Autodesk Fusion 360 part; units mm, degrees
(part 3 of 5)
  spline S734 degree 3 poles (4.2768, -3.4159) (4.27, -4.5634) (4.2456, -6.2234) (4.2225, -7.1047) knots 0 0 0 0 1 1 1 1
  spline S735 degree 3 poles (4.2225, -7.1047) (4.1736, -8.9658) (4.1741, -8.9676) (4.6986, -8.9676) knots 0 0 0 0 1 1 1 1
  spline S736 degree 3 poles (4.6986, -8.9676) (4.9293, -8.9676) (5.068, -8.9294) (5.1437, -8.8451) knots 0 0 0 0 1 1 1 1
  spline S737 degree 3 poles (-7.7375, -7.165) (-7.6403, -7.0562) (-7.6359, -6.8494) (-7.6984, -5.3274) knots 0 0 0 0 1 1 1 1
  spline S738 degree 3 poles (-7.6984, -5.3274) (-7.7797, -3.3444) (-7.7614, -3.2272) (-7.3703, -3.2272) knots 0 0 0 0 1 1 1 1
  spline S739 degree 3 poles (-7.3703, -3.2272) (-7.0455, -3.2272) (-6.9853, -3.3847) (-6.9853, -4.2336) knots 0 0 0 0 1 1 1 1
  spline S740 degree 3 poles (-6.9853, -4.2336) (-6.9853, -5.2382) (-7.167, -5.17) (-4.517, -5.1604) knots 0 0 0 0 1 1 1 1
  spline S741 degree 3 poles (-4.517, -5.1604) (-2.7083, -5.1538) (-2.2947, -5.1343) (-2.1944, -5.051) knots 0 0 0 0 1 1 1 1
  spline S742 degree 3 poles (-2.1944, -5.051) (-2.0819, -4.9577) (-2.0757, -4.8021) (-2.1141, -3.066) knots 0 0 0 0 1 1 1 1
  spline S743 degree 3 poles (-2.1141, -3.066) (-2.1371, -2.0299) (-2.1733, -1.154) (-2.1946, -1.1196) knots 0 0 0 0 1 1 1 1
  spline S744 degree 3 poles (-2.1946, -1.1196) (-2.2168, -1.0837) (-4.8195, -1.0571) (-8.3145, -1.0571) knots 0 0 0 0 1 1 1 1
  spline S745 degree 3 poles (-8.3145, -1.0571) (-13.6654, -1.0571) (-14.4085, -1.0699) (-14.5022, -1.1636) knots 0 0 0 0 1 1 1 1
  spline S746 degree 3 poles (-14.5022, -1.1636) (-14.6184, -1.2797) (-14.6146, -1.6645) (-14.4728, -4.1373) knots 0 0 0 0 1 1 1 1
  spline S747 degree 3 poles (-14.4728, -4.1373) (-14.3583, -6.1352) (-14.267, -6.958) (-14.1447, -7.0942) knots 0 0 0 0 1 1 1 1
  spline S748 degree 3 poles (-14.1447, -7.0942) (-14.0447, -7.2056) (-13.7867, -7.2176) (-11.1229, -7.235) knots 0 0 0 0 1 1 1 1
  spline S749 degree 3 poles (-11.1229, -7.235) (-9.521, -7.2455) (-8.1286, -7.2616) (-8.0287, -7.2708) knots 0 0 0 0 1 1 1 1
  spline S750 degree 3 poles (-8.0287, -7.2708) (-7.9262, -7.2802) (-7.7993, -7.2341) (-7.7375, -7.165) knots 0 0 0 0 1 1 1 1
  spline S751 degree 3 poles (-15.1497, -7.1114) (-15.0136, -6.9753) (-15.0146, -7.1038) (-15.1381, -5.6424) knots 0 0 0 0 1 1 1 1
  spline S752 degree 3 poles (-15.1381, -5.6424) (-15.1934, -4.9878) (-15.2581, -3.964) (-15.2817, -3.3672) knots 0 0 0 0 1 1 1 1
  spline S753 degree 3 poles (-15.2817, -3.3672) (-15.3054, -2.7704) (-15.3347, -2.0537) (-15.3469, -1.7744) knots 0 0 0 0 1 1 1 1
  spline S754 degree 3 poles (-15.3469, -1.7744) (-15.359, -1.4952) (-15.4081, -1.2196) (-15.4559, -1.1619) knots 0 0 0 0 1 1 1 1
  spline S755 degree 3 poles (-15.4559, -1.1619) (-15.5314, -1.071) (-16.0972, -1.0571) (-19.7322, -1.0571) knots 0 0 0 0 1 1 1 1
  spline S756 degree 3 poles (-19.7322, -1.0571) (-23.6509, -1.0571) (-23.9255, -1.065) (-23.9853, -1.1796) knots 0 0 0 0 1 1 1 1
  spline S757 degree 3 poles (-23.9853, -1.1796) (-24.1581, -1.5109) (-23.6522, -6.7547) (-23.4262, -6.9753) knots 0 0 0 0 1 1 1 1
  spline S758 degree 3 poles (-23.4262, -6.9753) (-23.3521, -7.0476) (-22.6326, -7.0805) (-20.1461, -7.1252) knots 0 0 0 0 1 1 1 1
  spline S759 degree 3 poles (-20.1461, -7.1252) (-18.3942, -7.1567) (-16.579, -7.1921) (-16.1123, -7.2039) knots 0 0 0 0 1 1 1 1
  spline S760 degree 3 poles (-16.1123, -7.2039) (-15.4022, -7.2219) (-15.2451, -7.2068) (-15.1497, -7.1114) knots 0 0 0 0 1 1 1 1
  spline S761 degree 3 poles (20.0321, -7.0477) (20.1165, -6.946) (20.2451, -5.9874) (20.3851, -4.4173) knots 0 0 0 0 1 1 1 1
  spline S762 degree 3 poles (20.3851, -4.4173) (20.4607, -3.5699) (20.47, -3.5361) (20.6793, -3.3497) knots 0 0 0 0 1 1 1 1
  spline S763 degree 3 poles (20.6793, -3.3497) (20.8909, -3.1612) (20.914, -3.1572) (21.7814, -3.1572) knots 0 0 0 0 1 1 1 1
  line L87 (21.7814, -3.1572) -> (22.6674, -3.1572)
  line L88 (22.6674, -3.1572) -> (22.9766, -3.4722)
  spline S764 degree 3 poles (22.9766, -3.4722) (23.2635, -3.7646) (23.3116, -3.7873) (23.6454, -3.7873) knots 0 0 0 0 1 1 1 1
  spline S765 degree 3 poles (23.6454, -3.7873) (24.1649, -3.7873) (24.2165, -3.7033) (24.269, -2.7722) knots 0 0 0 0 1 1 1 1
  spline S766 degree 3 poles (24.269, -2.7722) (24.2929, -2.3487) (24.3272, -1.8511) (24.3453, -1.6665) knots 0 0 0 0 1 1 1 1
  spline S767 degree 3 poles (24.3453, -1.6665) (24.4099, -1.008) (24.6837, -1.0571) (20.9465, -1.0571) knots 0 0 0 0 1 1 1 1
  spline S768 degree 3 poles (20.9465, -1.0571) (17.7701, -1.0571) (17.6588, -1.0616) (17.5887, -1.1925) knots 0 0 0 0 1 1 1 1
  spline S769 degree 3 poles (17.5887, -1.1925) (17.5489, -1.267) (17.516, -1.6371) (17.5157, -2.015) knots 0 0 0 0 1 1 1 1
  spline S770 degree 3 poles (17.5157, -2.015) (17.5149, -2.7862) (17.3457, -5.3852) (17.2344, -6.3324) knots 0 0 0 0 1 1 1 1
  spline S771 degree 3 poles (17.2344, -6.3324) (17.1803, -6.7925) (17.1824, -6.9776) (17.2425, -7.05) knots 0 0 0 0 1 1 1 1
  spline S772 degree 3 poles (17.2425, -7.05) (17.3623, -7.1943) (19.9121, -7.1922) (20.0321, -7.0477) knots 0 0 0 0 1 1 1 1
  spline S773 degree 3 poles (27.0719, -6.9725) (28.7644, -6.9359) (29.1939, -6.9073) (29.2848, -6.8252) knots 0 0 0 0 1 1 1 1
  spline S774 degree 3 poles (29.2848, -6.8252) (29.5576, -6.5788) (30.1767, -1.4027) (29.9641, -1.1465) knots 0 0 0 0 1 1 1 1
  spline S775 degree 3 poles (29.9641, -1.1465) (29.9066, -1.0773) (29.3748, -1.0573) (27.6058, -1.0582) knots 0 0 0 0 1 1 1 1
  spline S776 degree 3 poles (27.6058, -1.0582) (26.3464, -1.0587) (25.2763, -1.088) (25.2205, -1.1233) knots 0 0 0 0 1 1 1 1
  spline S777 degree 3 poles (25.2205, -1.1233) (25.1439, -1.1718) (25.1061, -1.4402) (25.0654, -2.2248) knots 0 0 0 0 1 1 1 1
  spline S778 degree 3 poles (25.0654, -2.2248) (25.0016, -3.4565) (24.8292, -5.2439) (24.686, -6.16) knots 0 0 0 0 1 1 1 1
  spline S779 degree 3 poles (24.686, -6.16) (24.5925, -6.7582) (24.5935, -6.8289) (24.6965, -6.9428) knots 0 0 0 0 1 1 1 1
  spline S780 degree 3 poles (24.6965, -6.9428) (24.7589, -7.0117) (24.8463, -7.0568) (24.8908, -7.043) knots 0 0 0 0 1 1 1 1
  spline S781 degree 3 poles (24.8908, -7.043) (24.9353, -7.0292) (25.9168, -6.9975) (27.0719, -6.9725) knots 0 0 0 0 1 1 1 1
  spline S782 degree 3 poles (-24.3456, -6.866) (-24.3039, -6.7882) (-24.2846, -6.7007) (-24.3025, -6.6717) knots 0 0 0 0 1 1 1 1
  spline S783 degree 3 poles (-24.3025, -6.6717) (-24.3372, -6.6155) (-24.5035, -5.3894) (-24.6286, -4.2679) knots 0 0 0 0 1 1 1 1
  spline S784 degree 3 poles (-24.6286, -4.2679) (-24.67, -3.8969) (-24.728, -3.0721) (-24.7576, -2.435) knots 0 0 0 0 1 1 1 1
  spline S785 degree 3 poles (-24.7576, -2.435) (-24.7937, -1.6576) (-24.8414, -1.2404) (-24.9025, -1.1668) knots 0 0 0 0 1 1 1 1
  spline S786 degree 3 poles (-24.9025, -1.1668) (-24.9817, -1.0713) (-25.2907, -1.0571) (-27.2926, -1.0571) knots 0 0 0 0 1 1 1 1
  spline S787 degree 3 poles (-27.2926, -1.0571) (-29.4108, -1.0571) (-29.5968, -1.0667) (-29.6566, -1.1796) knots 0 0 0 0 1 1 1 1
  spline S788 degree 3 poles (-29.6566, -1.1796) (-29.8456, -1.5361) (-29.2581, -6.514) (-28.9925, -6.8075) knots 0 0 0 0 1 1 1 1
  spline S789 degree 3 poles (-28.9925, -6.8075) (-28.871, -6.9417) (-28.7554, -6.9479) (-25.5564, -6.9919) knots 0 0 0 0 1 1 1 1
  spline S790 degree 3 poles (-25.5564, -6.9919) (-24.4807, -7.0066) (-24.4173, -7.0001) (-24.3456, -6.866) knots 0 0 0 0 1 1 1 1
  spline S791 degree 3 poles (-29.9974, -6.7448) (-29.8983, -6.6353) (-29.8967, -6.5674) (-29.9829, -6.115) knots 0 0 0 0 1 1 1 1
  spline S792 degree 3 poles (-29.9829, -6.115) (-30.1257, -5.3656) (-30.35, -3.4788) (-30.4384, -2.2838) knots 0 0 0 0 1 1 1 1
  spline S793 degree 3 poles (-30.4384, -2.2838) (-30.481, -1.7072) (-30.5492, -1.1953) (-30.5899, -1.1462) knots 0 0 0 0 1 1 1 1
  spline S794 degree 3 poles (-30.5899, -1.1462) (-30.6927, -1.0223) (-33.6594, -1.0176) (-33.7829, -1.1411) knots 0 0 0 0 1 1 1 1
  spline S795 degree 3 poles (-33.7829, -1.1411) (-33.9031, -1.2613) (-33.8872, -1.8592) (-33.7257, -3.2908) knots 0 0 0 0 1 1 1 1
  spline S796 degree 3 poles (-33.7257, -3.2908) (-33.5508, -4.8422) (-33.2687, -6.4463) (-33.1506, -6.5614) knots 0 0 0 0 1 1 1 1
  spline S797 degree 3 poles (-33.1506, -6.5614) (-33.0737, -6.6365) (-32.3628, -6.7147) (-30.7867, -6.8216) knots 0 0 0 0 1 1 1 1
  spline S798 degree 3 poles (-30.7867, -6.8216) (-30.6135, -6.8334) (-30.3899, -6.8485) (-30.29, -6.8552) knots 0 0 0 0 1 1 1 1
  spline S799 degree 3 poles (-30.29, -6.8552) (-30.1901, -6.8619) (-30.0584, -6.8122) (-29.9974, -6.7448) knots 0 0 0 0 1 1 1 1
  spline S800 degree 3 poles (31.1807, -6.7419) (31.275, -6.6475) (31.5379, -5.2425) (31.6615, -4.1723) knots 0 0 0 0 1 1 1 1
  spline S801 degree 3 poles (31.6615, -4.1723) (31.7475, -3.4274) (31.7585, -3.3948) (31.9975, -3.1747) knots 0 0 0 0 1 1 1 1
  line L89 (31.9975, -3.1747) -> (32.2445, -2.9472)
  line L90 (32.2445, -2.9472) -> (33.0281, -2.9472)
  spline S802 degree 3 poles (33.0281, -2.9472) (34.0757, -2.9472) (34.0873, -2.9374) (34.1613, -1.9839) knots 0 0 0 0 1 1 1 1
  spline S803 degree 3 poles (34.1613, -1.9839) (34.1919, -1.5888) (34.1907, -1.2186) (34.1586, -1.1613) knots 0 0 0 0 1 1 1 1
  spline S804 degree 3 poles (34.1586, -1.1613) (34.0766, -1.0147) (31.0188, -1.0054) (30.8728, -1.1513) knots 0 0 0 0 1 1 1 1
  spline S805 degree 3 poles (30.8728, -1.1513) (30.8151, -1.209) (30.7711, -1.4464) (30.7592, -1.7638) knots 0 0 0 0 1 1 1 1
  spline S806 degree 3 poles (30.7592, -1.7638) (30.7294, -2.5612) (30.4864, -4.8147) (30.3292, -5.7512) knots 0 0 0 0 1 1 1 1
  spline S807 degree 3 poles (30.3292, -5.7512) (30.1516, -6.8092) (30.1825, -6.8934) (30.732, -6.8498) knots 0 0 0 0 1 1 1 1
  spline S808 degree 3 poles (30.732, -6.8498) (30.9355, -6.8337) (31.1374, -6.7851) (31.1807, -6.7419) knots 0 0 0 0 1 1 1 1
  line L91 (31.1807, -6.7419) -> (31.1807, -6.7419)
  spline S809 degree 3 poles (33.4591, -6.5656) (33.5108, -6.5139) (33.6498, -5.8956) (33.768, -5.1916) knots 0 0 0 0 1 1 1 1
  spline S810 degree 3 poles (33.768, -5.1916) (33.9788, -3.9355) (33.9803, -3.9092) (33.8502, -3.7791) knots 0 0 0 0 1 1 1 1
  spline S811 degree 3 poles (33.8502, -3.7791) (33.7337, -3.6626) (33.6513, -3.6521) (33.1716, -3.6926) knots 0 0 0 0 1 1 1 1
  spline S812 degree 3 poles (33.1716, -3.6926) (32.8714, -3.718) (32.5872, -3.7772) (32.5402, -3.8242) knots 0 0 0 0 1 1 1 1
  spline S813 degree 3 poles (32.5402, -3.8242) (32.4932, -3.8713) (32.4163, -4.2051) (32.3693, -4.566) knots 0 0 0 0 1 1 1 1
  spline S814 degree 3 poles (32.3693, -4.566) (32.3223, -4.927) (32.2348, -5.5153) (32.1749, -5.8734) knots 0 0 0 0 1 1 1 1
  spline S815 degree 3 poles (32.1749, -5.8734) (32.0308, -6.7344) (32.051, -6.761) (32.8072, -6.7027) knots 0 0 0 0 1 1 1 1
  spline S816 degree 3 poles (32.8072, -6.7027) (33.1268, -6.678) (33.4052, -6.6195) (33.4591, -6.5656) knots 0 0 0 0 1 1 1 1
  spline S817 degree 3 poles (23.8843, -5.9952) (23.925, -5.9462) (23.9908, -5.6461) (24.0307, -5.3283) knots 0 0 0 0 1 1 1 1
  spline S818 degree 3 poles (24.0307, -5.3283) (24.123, -4.5919) (24.0582, -4.4907) (23.519, -4.5295) knots 0 0 0 0 1 1 1 1
  spline S819 degree 3 poles (23.519, -4.5295) (23.3207, -4.5438) (23.1213, -4.5953) (23.0758, -4.6439) knots 0 0 0 0 1 1 1 1
  spline S820 degree 3 poles (23.0758, -4.6439) (23.0304, -4.6925) (22.9593, -5.0001) (22.9177, -5.3274) knots 0 0 0 0 1 1 1 1
  spline S821 degree 3 poles (22.9177, -5.3274) (22.8494, -5.8659) (22.8539, -5.9324) (22.9659, -6.0277) knots 0 0 0 0 1 1 1 1
  spline S822 degree 3 poles (22.9659, -6.0277) (23.1151, -6.1546) (23.7713, -6.1315) (23.8843, -5.9952) knots 0 0 0 0 1 1 1 1
  spline S823 degree 3 poles (-28.6306, -0.203) (-28.578, -0.1505) (-28.5466, 0.1107) (-28.5466, 0.4945) knots 0 0 0 0 1 1 1 1
  spline S824 degree 3 poles (-28.5466, 0.4945) (-28.5466, 1.0295) (-28.5639, 1.1174) (-28.682, 1.1806) knots 0 0 0 0 1 1 1 1
  spline S825 degree 3 poles (-28.682, 1.1806) (-28.7669, 1.226) (-29.6198, 1.2531) (-30.9691, 1.2531) knots 0 0 0 0 1 1 1 1
  spline S826 degree 3 poles (-30.9691, 1.2531) (-33.5287, 1.2531) (-33.3769, 1.302) (-33.3769, 0.4772) knots 0 0 0 0 1 1 1 1
  spline S827 degree 3 poles (-33.3769, 0.4772) (-33.3769, 0.0758) (-33.348, -0.0959) (-33.2669, -0.177) knots 0 0 0 0 1 1 1 1
  spline S828 degree 3 poles (-33.2669, -0.177) (-33.1715, -0.2724) (-32.8616, -0.287) (-30.9357, -0.287) knots 0 0 0 0 1 1 1 1
  spline S829 degree 3 poles (-30.9357, -0.287) (-29.3015, -0.287) (-28.6924, -0.2648) (-28.6306, -0.203) knots 0 0 0 0 1 1 1 1
  spline S830 degree 3 poles (-19.6, -0.203) (-19.4866, -0.0896) (-19.4866, 1.0556) (-19.6, 1.1691) knots 0 0 0 0 1 1 1 1
  spline S831 degree 3 poles (-19.6, 1.1691) (-19.6634, 1.2324) (-20.6523, 1.2531) (-23.6213, 1.2531) knots 0 0 0 0 1 1 1 1
  line L92 (-23.6213, 1.2531) -> (-27.5586, 1.2531)
  line L93 (-27.5586, 1.2531) -> (-27.6676, 1.0975)
  spline S832 degree 3 poles (-27.6676, 1.0975) (-27.7408, 0.9929) (-27.7765, 0.7824) (-27.7765, 0.4554) knots 0 0 0 0 1 1 1 1
  spline S833 degree 3 poles (-27.7765, 0.4554) (-27.7765, -0.3571) (-28.1691, -0.287) (-23.6144, -0.287) knots 0 0 0 0 1 1 1 1
  spline S834 degree 3 poles (-23.6144, -0.287) (-20.6508, -0.287) (-19.6634, -0.2664) (-19.6, -0.203) knots 0 0 0 0 1 1 1 1
  spline S835 degree 3 poles (-4.1031, -0.1712) (-3.9171, -0.0028) (-3.9167, 0.9685) (-4.1026, 1.1368) knots 0 0 0 0 1 1 1 1
  spline S836 degree 3 poles (-4.1026, 1.1368) (-4.2193, 1.2424) (-4.8358, 1.2521) (-11.382, 1.2517) knots 0 0 0 0 1 1 1 1
  line L94 (-11.382, 1.2517) -> (-18.5339, 1.2512)
  line L95 (-18.5339, 1.2512) -> (-18.6402, 1.0889)
  spline S837 degree 3 poles (-18.6402, 1.0889) (-18.7826, 0.8717) (-18.7685, 0.0077) (-18.6199, -0.1645) knots 0 0 0 0 1 1 1 1
  spline S838 degree 3 poles (-18.6199, -0.1645) (-18.5205, -0.2797) (-18.0872, -0.287) (-11.3726, -0.287) knots 0 0 0 0 1 1 1 1
  spline S839 degree 3 poles (-11.3726, -0.287) (-4.8256, -0.287) (-4.2204, -0.2774) (-4.103, -0.1712) knots 0 0 0 0 1 1 1 1
  line L96 (-4.103, -0.1712) -> (-4.1031, -0.1712)
  spline S840 degree 3 poles (13.232, -0.203) (13.3455, -0.0896) (13.3455, 1.0556) (13.232, 1.1691) knots 0 0 0 0 1 1 1 1
  spline S841 degree 3 poles (13.232, 1.1691) (13.1062, 1.2948) (-3.0167, 1.2906) (-3.1211, 1.1648) knots 0 0 0 0 1 1 1 1
  spline S842 degree 3 poles (-3.1211, 1.1648) (-3.2358, 1.0267) (-3.2513, -0.042) (-3.1405, -0.1754) knots 0 0 0 0 1 1 1 1
  spline S843 degree 3 poles (-3.1405, -0.1754) (-3.0567, -0.2764) (-2.2771, -0.287) (5.0501, -0.287) knots 0 0 0 0 1 1 1 1
  spline S844 degree 3 poles (5.0501, -0.287) (11.2551, -0.287) (13.1676, -0.2674) (13.232, -0.203) knots 0 0 0 0 1 1 1 1
  spline S845 degree 3 poles (20.2324, -0.203) (20.2847, -0.1507) (20.3164, 0.1081) (20.3164, 0.483) knots 0 0 0 0 1 1 1 1
  spline S846 degree 3 poles (20.3164, 0.483) (20.3164, 0.8579) (20.2847, 1.1167) (20.2324, 1.1691) knots 0 0 0 0 1 1 1 1
  spline S847 degree 3 poles (20.2324, 1.1691) (20.1698, 1.2317) (19.4099, 1.2531) (17.2453, 1.2531) knots 0 0 0 0 1 1 1 1
  spline S848 degree 3 poles (17.2453, 1.2531) (13.8367, 1.2531) (14.0861, 1.3129) (14.0861, 0.4952) knots 0 0 0 0 1 1 1 1
  spline S849 degree 3 poles (14.0861, 0.4952) (14.0861, -0.3526) (13.8223, -0.287) (17.2331, -0.287) knots 0 0 0 0 1 1 1 1
  spline S850 degree 3 poles (17.2331, -0.287) (19.4072, -0.287) (20.1698, -0.2657) (20.2324, -0.203) knots 0 0 0 0 1 1 1 1
  spline S851 degree 3 poles (28.0989, -0.1712) (28.2013, -0.0785) (28.2269, 0.05) (28.2269, 0.4708) knots 0 0 0 0 1 1 1 1
  spline S852 degree 3 poles (28.2269, 0.4708) (28.2269, 1.3245) (28.5557, 1.2531) (24.6249, 1.2531) knots 0 0 0 0 1 1 1 1
  spline S853 degree 3 poles (24.6249, 1.2531) (22.0968, 1.2531) (21.2335, 1.2321) (21.1705, 1.1691) knots 0 0 0 0 1 1 1 1
  spline S854 degree 3 poles (21.1705, 1.1691) (21.1182, 1.1167) (21.0865, 0.8579) (21.0865, 0.483) knots 0 0 0 0 1 1 1 1
  spline S855 degree 3 poles (21.0865, 0.483) (21.0865, 0.1081) (21.1182, -0.1507) (21.1705, -0.203) knots 0 0 0 0 1 1 1 1
  spline S856 degree 3 poles (21.1705, -0.203) (21.2335, -0.266) (22.0941, -0.287) (24.6127, -0.287) knots 0 0 0 0 1 1 1 1
  spline S857 degree 3 poles (24.6127, -0.287) (27.6393, -0.287) (27.9835, -0.2756) (28.0989, -0.1712) knots 0 0 0 0 1 1 1 1
  spline S858 degree 3 poles (33.5592, -0.1712) (33.6616, -0.0785) (33.6873, 0.05) (33.6873, 0.4708) knots 0 0 0 0 1 1 1 1
  spline S859 degree 3 poles (33.6873, 0.4708) (33.6873, 1.3036) (33.8403, 1.2531) (31.3193, 1.2531) knots 0 0 0 0 1 1 1 1
  spline S860 degree 3 poles (31.3193, 1.2531) (28.7831, 1.2531) (28.927, 1.2986) (28.927, 0.4952) knots 0 0 0 0 1 1 1 1
  spline S861 degree 3 poles (28.927, 0.4952) (28.927, -0.3376) (28.774, -0.287) (31.295, -0.287) knots 0 0 0 0 1 1 1 1
  spline S862 degree 3 poles (31.295, -0.287) (33.1845, -0.287) (33.446, -0.2737) (33.5592, -0.1712) knots 0 0 0 0 1 1 1 1
  spline S863 degree 3 poles (22.4173, 2.1644) (22.4596, 2.2435) (22.46, 2.6704) (22.4183, 3.3284) knots 0 0 0 0 1 1 1 1
  line L97 (22.4183, 3.3284) -> (22.3525, 4.3676)
  line L98 (22.3525, 4.3676) -> (22.5733, 4.5954)
  spline S864 degree 3 poles (22.5733, 4.5954) (22.7891, 4.8181) (22.808, 4.8233) (23.4019, 4.8233) knots 0 0 0 0 1 1 1 1
  spline S865 degree 3 poles (23.4019, 4.8233) (23.8371, 4.8233) (24.0327, 4.8511) (24.0909, 4.9212) knots 0 0 0 0 1 1 1 1
  spline S866 degree 3 poles (24.0909, 4.9212) (24.2074, 5.0616) (24.1117, 5.9094) (23.9648, 6.037) knots 0 0 0 0 1 1 1 1
  spline S867 degree 3 poles (23.9648, 6.037) (23.8721, 6.1177) (23.1892, 6.1423) (20.1678, 6.1741) knots 0 0 0 0 1 1 1 1
  spline S868 degree 3 poles (20.1678, 6.1741) (17.4864, 6.2023) (16.4623, 6.1914) (16.405, 6.1341) knots 0 0 0 0 1 1 1 1
  spline S869 degree 3 poles (16.405, 6.1341) (16.3617, 6.0908) (16.3263, 5.846) (16.3263, 5.5902) knots 0 0 0 0 1 1 1 1
  spline S870 degree 3 poles (16.3263, 5.5902) (16.3263, 4.9083) (16.3284, 4.9073) (17.7234, 4.8861) knots 0 0 0 0 1 1 1 1
  line L99 (17.7234, 4.8861) -> (18.8755, 4.8686)
  line L100 (18.8755, 4.8686) -> (19.1134, 4.6505)
  line L101 (19.1134, 4.6505) -> (19.3513, 4.4325)
  line L102 (19.3513, 4.4325) -> (19.388, 3.3503)
  spline S871 degree 3 poles (19.388, 3.3503) (19.4082, 2.7551) (19.4528, 2.2137) (19.4872, 2.1472) knots 0 0 0 0 1 1 1 1
  spline S872 degree 3 poles (19.4872, 2.1472) (19.5425, 2.0401) (19.7011, 2.024) (20.8607, 2.0071) knots 0 0 0 0 1 1 1 1
  spline S873 degree 3 poles (20.8607, 2.0071) (21.5817, 1.9967) (22.2119, 1.9997) (22.2611, 2.0138) knots 0 0 0 0 1 1 1 1
  spline S874 degree 3 poles (22.2611, 2.0138) (22.3103, 2.028) (22.3806, 2.0958) (22.4174, 2.1644) knots 0 0 0 0 1 1 1 1
  line L103 (22.4174, 2.1644) -> (22.4173, 2.1644)
  spline S875 degree 3 poles (34.1084, 2.1407) (34.2143, 2.2533) (34.221, 2.3495) (34.166, 2.9682) knots 0 0 0 0 1 1 1 1
  spline S876 degree 3 poles (34.166, 2.9682) (34.0827, 3.9038) (34.0917, 3.8969) (32.9358, 3.9057) knots 0 0 0 0 1 1 1 1
  spline S877 degree 3 poles (32.9358, 3.9057) (32.4443, 3.9094) (31.6422, 3.9328) (31.1534, 3.9575) knots 0 0 0 0 1 1 1 1
  spline S878 degree 3 poles (31.1534, 3.9575) (30.2969, 4.0009) (30.2579, 4.0097) (30.0759, 4.1996) knots 0 0 0 0 1 1 1 1
  spline S879 degree 3 poles (30.0759, 4.1996) (29.9048, 4.3783) (29.8748, 4.4938) (29.7558, 5.4326) knots 0 0 0 0 1 1 1 1
  spline S880 degree 3 poles (29.7558, 5.4326) (29.5711, 6.8889) (29.4243, 7.6385) (29.2958, 7.781) knots 0 0 0 0 1 1 1 1
  spline S881 degree 3 poles (29.2958, 7.781) (29.1413, 7.9523) (28.5701, 7.9493) (28.4137, 7.7764) knots 0 0 0 0 1 1 1 1
  spline S882 degree 3 poles (28.4137, 7.7764) (28.3095, 7.6613) (28.308, 7.6004) (28.3979, 7.1289) knots 0 0 0 0 1 1 1 1
  spline S883 degree 3 poles (28.3979, 7.1289) (28.4524, 6.8426) (28.5523, 6.1265) (28.6199, 5.5376) knots 0 0 0 0 1 1 1 1
  line L104 (28.6199, 5.5376) -> (28.7428, 4.4668)
  line L105 (28.7428, 4.4668) -> (28.5185, 4.2425)
  line L106 (28.5185, 4.2425) -> (28.2942, 4.0182)
  line L107 (28.2942, 4.0182) -> (25.7929, 4.0419)
  spline S884 degree 3 poles (25.7929, 4.0419) (23.4252, 4.0643) (23.2876, 4.0587) (23.2157, 3.9369) knots 0 0 0 0 1 1 1 1
  spline S885 degree 3 poles (23.2157, 3.9369) (23.0937, 3.7299) (23.192, 2.1733) (23.3336, 2.0699) knots 0 0 0 0 1 1 1 1
  spline S886 degree 3 poles (23.3336, 2.0699) (23.417, 2.009) (24.7902, 1.9913) (28.717, 2.0007) knots 0 0 0 0 1 1 1 1
  spline S887 degree 3 poles (28.717, 2.0007) (33.7156, 2.0126) (33.9947, 2.0198) (34.1084, 2.1407) knots 0 0 0 0 1 1 1 1
  spline S888 degree 3 poles (-26.8081, 2.1141) (-26.7666, 2.1641) (-26.6984, 2.6918) (-26.6565, 3.2867) knots 0 0 0 0 1 1 1 1
  spline S889 degree 3 poles (-26.6565, 3.2867) (-26.5527, 4.7638) (-26.4054, 6.1913) (-26.2711, 7.0222) knots 0 0 0 0 1 1 1 1
  spline S890 degree 3 poles (-26.2711, 7.0222) (-26.123, 7.9391) (-26.1054, 7.9221) (-27.192, 7.9108) knots 0 0 0 0 1 1 1 1
  spline S891 degree 3 poles (-27.192, 7.9108) (-28.2199, 7.9001) (-29.2313, 7.8545) (-31.3456, 7.7237) knots 0 0 0 0 1 1 1 1
  spline S892 degree 3 poles (-31.3456, 7.7237) (-32.7876, 7.6344) (-33.0059, 7.6056) (-33.123, 7.4884) knots 0 0 0 0 1 1 1 1
  spline S893 degree 3 poles (-33.123, 7.4884) (-33.3262, 7.2852) (-33.6509, 5.1938) (-33.8931, 2.5274) knots 0 0 0 0 1 1 1 1
  spline S894 degree 3 poles (-33.8931, 2.5274) (-33.9414, 1.9957) (-34.1365, 2.0231) (-30.3003, 2.0231) knots 0 0 0 0 1 1 1 1
  spline S895 degree 3 poles (-30.3003, 2.0231) (-27.5829, 2.0231) (-26.8682, 2.0417) (-26.8081, 2.1141) knots 0 0 0 0 1 1 1 1
  spline S896 degree 3 poles (-21.1271, 2.1269) (-21.0745, 2.1903) (-21.0284, 2.5509) (-21.0087, 3.0545) knots 0 0 0 0 1 1 1 1
  spline S897 degree 3 poles (-21.0087, 3.0545) (-20.9909, 3.5075) (-20.9334, 4.3507) (-20.8808, 4.9283) knots 0 0 0 0 1 1 1 1
  spline S898 degree 3 poles (-20.8808, 4.9283) (-20.8029, 5.783) (-20.8019, 5.9954) (-20.875, 6.0702) knots 0 0 0 0 1 1 1 1
  spline S899 degree 3 poles (-20.875, 6.0702) (-20.9244, 6.1207) (-21.218, 6.2498) (-21.5275, 6.3569) knots 0 0 0 0 1 1 1 1
  spline S900 degree 3 poles (-21.5275, 6.3569) (-22.4234, 6.6671) (-23.1908, 7.1243) (-23.8563, 7.7441) knots 0 0 0 0 1 1 1 1
  spline S901 degree 3 poles (-23.8563, 7.7441) (-24.0886, 7.9604) (-24.1292, 7.9723) (-24.6388, 7.9729) knots 0 0 0 0 1 1 1 1
  spline S902 degree 3 poles (-24.6388, 7.9729) (-25.0146, 7.9733) (-25.2068, 7.9431) (-25.2774, 7.8724) knots 0 0 0 0 1 1 1 1
  spline S903 degree 3 poles (-25.2774, 7.8724) (-25.5207, 7.6291) (-26.0597, 2.4868) (-25.8775, 2.1465) knots 0 0 0 0 1 1 1 1
  spline S904 degree 3 poles (-25.8775, 2.1465) (-25.8165, 2.0325) (-25.637, 2.0231) (-23.5124, 2.0231) knots 0 0 0 0 1 1 1 1
  spline S905 degree 3 poles (-23.5124, 2.0231) (-21.5661, 2.0231) (-21.2, 2.039) (-21.1271, 2.1269) knots 0 0 0 0 1 1 1 1
  spline S906 degree 3 poles (-9.7877, 2.1253) (-9.6924, 2.2403) (-9.6684, 2.6014) (-9.6131, 4.7533) knots 0 0 0 0 1 1 1 1
  spline S907 degree 3 poles (-9.6131, 4.7533) (-9.5919, 5.5811) (-9.5545, 6.6089) (-9.5302, 7.0373) knots 0 0 0 0 1 1 1 1
  spline S908 degree 3 poles (-9.5302, 7.0373) (-9.5058, 7.4657) (-9.5066, 7.8988) (-9.532, 7.9998) knots 0 0 0 0 1 1 1 1
  line L108 (-9.532, 7.9998) -> (-9.5781, 8.1835)
  line L109 (-9.5781, 8.1835) -> (-10.9843, 8.1835)
  line L110 (-10.9843, 8.1835) -> (-12.3905, 8.1835)
  line L111 (-12.3905, 8.1835) -> (-13.1502, 7.7258)
  spline S909 degree 3 poles (-13.1502, 7.7258) (-15.0654, 6.5718) (-16.851, 6.0216) (-18.851, 5.9689) knots 0 0 0 0 1 1 1 1
  spline S910 degree 3 poles (-18.851, 5.9689) (-19.6852, 5.947) (-19.9174, 5.9194) (-19.9805, 5.835) knots 0 0 0 0 1 1 1 1
  spline S911 degree 3 poles (-19.9805, 5.835) (-20.119, 5.6496) (-20.3179, 2.3674) (-20.2041, 2.1456) knots 0 0 0 0 1 1 1 1
  spline S912 degree 3 poles (-20.2041, 2.1456) (-20.1451, 2.0306) (-19.8261, 2.0231) (-15.0069, 2.0231) knots 0 0 0 0 1 1 1 1
  spline S913 degree 3 poles (-15.0069, 2.0231) (-10.5907, 2.0231) (-9.8608, 2.0374) (-9.7878, 2.1253) knots 0 0 0 0 1 1 1 1
  line L112 (-9.7878, 2.1253) -> (-9.7877, 2.1253)
  spline S914 degree 3 poles (1.6085, 5.0269) (1.6255, 7.7783) (1.6178, 8.0058) (1.5035, 8.1321) knots 0 0 0 0 1 1 1 1
  spline S915 degree 3 poles (1.5035, 8.1321) (1.3831, 8.2653) (1.266, 8.2678) (-3.5658, 8.2402) knots 0 0 0 0 1 1 1 1
  spline S916 degree 3 poles (-3.5658, 8.2402) (-7.2678, 8.219) (-8.5372, 8.1908) (-8.6128, 8.1281) knots 0 0 0 0 1 1 1 1
  spline S917 degree 3 poles (-8.6128, 8.1281) (-8.7257, 8.0344) (-8.7633, 7.4807) (-8.8769, 4.241) knots 0 0 0 0 1 1 1 1
  spline S918 degree 3 poles (-8.8769, 4.241) (-8.9238, 2.9036) (-8.9224, 2.2511) (-8.8726, 2.1579) knots 0 0 0 0 1 1 1 1
  spline S919 degree 3 poles (-8.8726, 2.1579) (-8.8016, 2.0253) (-8.6826, 2.0226) (-3.6048, 2.0402) knots 0 0 0 0 1 1 1 1
  line L113 (-3.6048, 2.0402) -> (1.5903, 2.0581)
  line L114 (1.5903, 2.0581) -> (1.6085, 5.0269)
  spline S920 degree 3 poles (18.6197, 2.1106) (18.6631, 2.1645) (18.6762, 2.527) (18.6538, 3.0534) knots 0 0 0 0 1 1 1 1
  spline S921 degree 3 poles (18.6538, 3.0534) (18.6251, 3.7257) (18.5926, 3.9311) (18.5021, 4.013) knots 0 0 0 0 1 1 1 1
  spline S922 degree 3 poles (18.5021, 4.013) (18.4037, 4.1021) (17.8885, 4.1187) (14.968, 4.127) knots 0 0 0 0 1 1 1 1
  line L115 (14.968, 4.127) -> (11.5491, 4.1367)
  line L116 (11.5491, 4.1367) -> (11.2957, 4.369)
  line L117 (11.2957, 4.369) -> (11.0422, 4.6013)
  line L118 (11.0422, 4.6013) -> (11.0171, 5.4298)
  spline S923 degree 3 poles (11.0171, 5.4298) (10.9981, 6.0529) (10.9649, 6.2888) (10.883, 6.3809) knots 0 0 0 0 1 1 1 1
  spline S924 degree 3 poles (10.883, 6.3809) (10.7824, 6.4941) (10.5355, 6.5034) (7.6138, 6.5034) knots 0 0 0 0 1 1 1 1
  spline S925 degree 3 poles (7.6138, 6.5034) (5.2491, 6.5034) (4.4323, 6.4823) (4.3695, 6.4194) knots 0 0 0 0 1 1 1 1
  spline S926 degree 3 poles (4.3695, 6.4194) (4.3233, 6.3732) (4.285, 6.1763) (4.2844, 5.9819) knots 0 0 0 0 1 1 1 1
  spline S927 degree 3 poles (4.2844, 5.9819) (4.2831, 5.4971) (4.1645, 5.2839) (3.8813, 5.2564) knots 0 0 0 0 1 1 1 1
  spline S928 degree 3 poles (3.8813, 5.2564) (3.5685, 5.226) (3.5438, 5.3244) (3.4919, 6.8096) knots 0 0 0 0 1 1 1 1
  spline S929 degree 3 poles (3.4919, 6.8096) (3.465, 7.5816) (3.4176, 8.0977) (3.3682, 8.1571) knots 0 0 0 0 1 1 1 1
  spline S930 degree 3 poles (3.3682, 8.1571) (3.2729, 8.272) (2.727, 8.2861) (2.5268, 8.1789) knots 0 0 0 0 1 1 1 1
  spline S931 degree 3 poles (2.5268, 8.1789) (2.3907, 8.1061) (2.3877, 8.0345) (2.3993, 5.1512) knots 0 0 0 0 1 1 1 1
  spline S932 degree 3 poles (2.3993, 5.1512) (2.4068, 3.2866) (2.4372, 2.1659) (2.4818, 2.1106) knots 0 0 0 0 1 1 1 1
  spline S933 degree 3 poles (2.4818, 2.1106) (2.5376, 2.0415) (4.2365, 2.0231) (10.5508, 2.0231) knots 0 0 0 0 1 1 1 1
  spline S934 degree 3 poles (10.5508, 2.0231) (16.8652, 2.0231) (18.564, 2.0415) (18.6197, 2.1106) knots 0 0 0 0 1 1 1 1
  spline S935 degree 3 poles (27.8342, 4.8848) (27.9465, 5.0088) (27.943, 5.0877) (27.7727, 6.2674) knots 0 0 0 0 1 1 1 1
  spline S936 degree 3 poles (27.7727, 6.2674) (27.5422, 7.8648) (27.5383, 7.8746) (27.1107, 7.9314) knots 0 0 0 0 1 1 1 1
  spline S937 degree 3 poles (27.1107, 7.9314) (26.7193, 7.9833) (26.568, 7.9405) (26.5113, 7.7618) knots 0 0 0 0 1 1 1 1
  spline S938 degree 3 poles (26.5113, 7.7618) (26.4888, 7.691) (26.5348, 7.1505) (26.6135, 6.5607) knots 0 0 0 0 1 1 1 1
  spline S939 degree 3 poles (26.6135, 6.5607) (26.6921, 5.9709) (26.7742, 5.355) (26.7958, 5.192) knots 0 0 0 0 1 1 1 1
  spline S940 degree 3 poles (26.7958, 5.192) (26.8423, 4.841) (26.9555, 4.7583) (27.3935, 4.7554) knots 0 0 0 0 1 1 1 1
  spline S941 degree 3 poles (27.3935, 4.7554) (27.6213, 4.7539) (27.7499, 4.7917) (27.8342, 4.8848) knots 0 0 0 0 1 1 1 1
  spline S942 degree 3 poles (25.9775, 4.9171) (26.0906, 5.0534) (25.7938, 7.5275) (25.6255, 7.851) knots 0 0 0 0 1 1 1 1
  spline S943 degree 3 poles (25.6255, 7.851) (25.5759, 7.9464) (25.4714, 7.9735) (25.1528, 7.9735) knots 0 0 0 0 1 1 1 1
  spline S944 degree 3 poles (25.1528, 7.9735) (24.6167, 7.9735) (24.5566, 7.901) (24.6495, 7.3664) knots 0 0 0 0 1 1 1 1
  spline S945 degree 3 poles (24.6495, 7.3664) (24.6885, 7.142) (24.7699, 6.5196) (24.8304, 5.9833) knots 0 0 0 0 1 1 1 1
  spline S946 degree 3 poles (24.8304, 5.9833) (24.8909, 5.447) (24.9749, 4.9666) (25.0171, 4.9158) knots 0 0 0 0 1 1 1 1
  spline S947 degree 3 poles (25.0171, 4.9158) (25.1211, 4.7905) (25.8733, 4.7916) (25.9775, 4.9171) knots 0 0 0 0 1 1 1 1
  spline S948 degree 3 poles (13.8751, 4.9972) (13.9663, 5.107) (13.941, 5.8339) (13.7973, 7.235) knots 0 0 0 0 1 1 1 1
  spline S949 degree 3 poles (13.7973, 7.235) (13.7088, 8.0986) (13.6674, 8.1835) (13.3344, 8.1835) knots 0 0 0 0 1 1 1 1
  spline S950 degree 3 poles (13.3344, 8.1835) (12.9522, 8.1835) (12.616, 8.5288) (12.616, 8.9211) knots 0 0 0 0 1 1 1 1
  spline S951 degree 3 poles (12.616, 8.9211) (12.616, 9.0807) (12.582, 9.4762) (12.5404, 9.8) knots 0 0 0 0 1 1 1 1
  spline S952 degree 3 poles (12.5404, 9.8) (12.4319, 10.6454) (12.4535, 10.6337) (11.0121, 10.6337) knots 0 0 0 0 1 1 1 1
  spline S953 degree 3 poles (11.0121, 10.6337) (10.1968, 10.6337) (9.8184, 10.6083) (9.7598, 10.5496) knots 0 0 0 0 1 1 1 1
  spline S954 degree 3 poles (9.7598, 10.5496) (9.7069, 10.4968) (9.6758, 10.2327) (9.6758, 9.8376) knots 0 0 0 0 1 1 1 1
  spline S955 degree 3 poles (9.6758, 9.8376) (9.6758, 8.9934) (9.7134, 8.9535) (10.5118, 8.9535) knots 0 0 0 0 1 1 1 1
  spline S956 degree 3 poles (10.5118, 8.9535) (11.0693, 8.9535) (11.1341, 8.9385) (11.3479, 8.76) knots 0 0 0 0 1 1 1 1
  line L119 (11.3479, 8.76) -> (11.5797, 8.5665)
  line L120 (11.5797, 8.5665) -> (11.6862, 6.8524)
  spline S957 degree 3 poles (11.6862, 6.8524) (11.7687, 5.5257) (11.817, 5.1106) (11.9002, 5.0158) knots 0 0 0 0 1 1 1 1
  spline S958 degree 3 poles (11.9002, 5.0158) (11.9919, 4.9112) (12.1376, 4.8933) (12.8983, 4.8933) knots 0 0 0 0 1 1 1 1
  spline S959 degree 3 poles (12.8983, 4.8933) (13.6002, 4.8933) (13.8072, 4.9153) (13.8751, 4.9972) knots 0 0 0 0 1 1 1 1
  spline S960 degree 3 poles (15.5068, 5.0175) (15.6098, 5.1313) (15.61, 5.2576) (15.5084, 6.5401) knots 0 0 0 0 1 1 1 1
  spline S961 degree 3 poles (15.5084, 6.5401) (15.427, 7.5675) (15.3693, 7.971) (15.291, 8.061) knots 0 0 0 0 1 1 1 1
  spline S962 degree 3 poles (15.291, 8.061) (15.1481, 8.2252) (14.7699, 8.2191) (14.617, 8.0501) knots 0 0 0 0 1 1 1 1
  spline S963 degree 3 poles (14.617, 8.0501) (14.503, 7.9241) (14.5028, 7.8379) (14.6131, 6.4925) knots 0 0 0 0 1 1 1 1
  spline S964 degree 3 poles (14.6131, 6.4925) (14.6773, 5.7092) (14.7621, 5.0289) (14.8016, 4.9808) knots 0 0 0 0 1 1 1 1
  spline S965 degree 3 poles (14.8016, 4.9808) (14.9102, 4.8481) (15.3754, 4.8723) (15.5068, 5.0175) knots 0 0 0 0 1 1 1 1
  spline S966 degree 3 poles (-18.3144, 6.8009) (-18.1828, 6.9072) (-18.0354, 7.2779) (-17.7273, 8.2779) knots 0 0 0 0 1 1 1 1
  spline S967 degree 3 poles (-17.7273, 8.2779) (-17.5362, 8.8982) (-17.5085, 9.0617) (-17.5765, 9.1704) knots 0 0 0 0 1 1 1 1
  spline S968 degree 3 poles (-17.5765, 9.1704) (-17.7551, 9.4565) (-17.8188, 9.3908) (-18.7541, 7.9565) knots 0 0 0 0 1 1 1 1
  spline S969 degree 3 poles (-18.7541, 7.9565) (-19.2888, 7.1366) (-19.3704, 6.9737) (-19.3063, 6.8539) knots 0 0 0 0 1 1 1 1
  spline S970 degree 3 poles (-19.3063, 6.8539) (-19.2443, 6.7381) (-19.1599, 6.7134) (-18.8269, 6.7134) knots 0 0 0 0 1 1 1 1
  spline S971 degree 3 poles (-18.8269, 6.7134) (-18.6046, 6.7134) (-18.374, 6.7528) (-18.3144, 6.8009) knots 0 0 0 0 1 1 1 1
  spline S972 degree 3 poles (-20.4601, 6.8985) (-20.3955, 6.9233) (-20.0006, 7.4637) (-19.5826, 8.0994) knots 0 0 0 0 1 1 1 1
  spline S973 degree 3 poles (-19.5826, 8.0994) (-18.9726, 9.0271) (-18.836, 9.2801) (-18.8901, 9.3812) knots 0 0 0 0 1 1 1 1
  spline S974 degree 3 poles (-18.8901, 9.3812) (-18.9271, 9.4504) (-19.1599, 9.6037) (-19.4073, 9.7218) knots 0 0 0 0 1 1 1 1
  spline S975 degree 3 poles (-19.4073, 9.7218) (-19.9721, 9.9914) (-20.4937, 10.4006) (-20.7912, 10.8077) knots 0 0 0 0 1 1 1 1
  spline S976 degree 3 poles (-20.7912, 10.8077) (-20.9176, 10.9808) (-21.0891, 11.1411) (-21.1723, 11.164) knots 0 0 0 0 1 1 1 1
  spline S977 degree 3 poles (-21.1723, 11.164) (-21.2707, 11.1911) (-21.6002, 11.0844) (-22.1173, 10.8579) knots 0 0 0 0 1 1 1 1
  spline S978 degree 3 poles (-22.1173, 10.8579) (-22.554, 10.6666) (-23.1318, 10.4265) (-23.4013, 10.3244) knots 0 0 0 0 1 1 1 1
  spline S979 degree 3 poles (-23.4013, 10.3244) (-24.1514, 10.04) (-24.3472, 9.9427) (-24.3892, 9.8334) knots 0 0 0 0 1 1 1 1
  spline S980 degree 3 poles (-24.3892, 9.8334) (-24.4843, 9.5856) (-23.5278, 8.3981) (-22.807, 7.8691) knots 0 0 0 0 1 1 1 1
  spline S981 degree 3 poles (-22.807, 7.8691) (-22.3712, 7.5492) (-21.697, 7.2163) (-21.0911, 7.022) knots 0 0 0 0 1 1 1 1
  spline S982 degree 3 poles (-21.0911, 7.022) (-20.8216, 6.9355) (-20.5958, 6.8622) (-20.5893, 6.8591) knots 0 0 0 0 1 1 1 1
  spline S983 degree 3 poles (-20.5893, 6.8591) (-20.5828, 6.856) (-20.5247, 6.8737) (-20.4601, 6.8985) knots 0 0 0 0 1 1 1 1
  spline S984 degree 3 poles (23.8373, 6.9942) (23.9203, 7.1127) (23.922, 7.2207) (23.848, 7.6767) knots 0 0 0 0 1 1 1 1
  line L121 (23.848, 7.6767) -> (23.76, 8.2185)
  line L122 (23.76, 8.2185) -> (23.9533, 8.4635)
  spline S985 degree 3 poles (23.9533, 8.4635) (24.1423, 8.7031) (24.159, 8.709) (24.7103, 8.7287) knots 0 0 0 0 1 1 1 1
  spline S986 degree 3 poles (24.7103, 8.7287) (25.4385, 8.7549) (25.4793, 8.7986) (25.3639, 9.4295) knots 0 0 0 0 1 1 1 1
  spline S987 degree 3 poles (25.3639, 9.4295) (25.2104, 10.269) (24.8575, 11.6449) (24.7543, 11.8062) knots 0 0 0 0 1 1 1 1
  spline S988 degree 3 poles (24.7543, 11.8062) (24.625, 12.0082) (24.1753, 12.0267) (24.0037, 11.837) knots 0 0 0 0 1 1 1 1
  spline S989 degree 3 poles (24.0037, 11.837) (23.8983, 11.7205) (23.8978, 11.6602) (23.9978, 11.0873) knots 0 0 0 0 1 1 1 1
  spline S990 degree 3 poles (23.9978, 11.0873) (24.0576, 10.7447) (24.1195, 10.4434) (24.1353, 10.4177) knots 0 0 0 0 1 1 1 1
  spline S991 degree 3 poles (24.1353, 10.4177) (24.1512, 10.3921) (24.07, 10.2412) (23.955, 10.0824) knots 0 0 0 0 1 1 1 1
  line L123 (23.955, 10.0824) -> (23.7458, 9.7936)
  line L124 (23.7458, 9.7936) -> (22.8875, 9.7936)
  line L125 (22.8875, 9.7936) -> (22.0292, 9.7936)
  line L126 (22.0292, 9.7936) -> (21.669, 10.1086)
  line L127 (21.669, 10.1086) -> (21.3089, 10.4236)
  line L128 (21.3089, 10.4236) -> (19.1762, 10.4236)
  spline S992 degree 3 poles (19.1762, 10.4236) (17.4235, 10.4236) (17.0288, 10.406) (16.9612, 10.3246) knots 0 0 0 0 1 1 1 1
  spline S993 degree 3 poles (16.9612, 10.3246) (16.8981, 10.2486) (16.9045, 10.0434) (16.989, 9.4374) knots 0 0 0 0 1 1 1 1
  line L129 (16.989, 9.4374) -> (17.099, 8.649)
  line L130 (17.099, 8.649) -> (16.9051, 8.4349)
  spline S994 degree 3 poles (16.9051, 8.4349) (16.6606, 8.1648) (16.5915, 8.1143) (16.5235, 8.1563) knots 0 0 0 0 1 1 1 1
  spline S995 degree 3 poles (16.5235, 8.1563) (16.4936, 8.1748) (16.4055, 8.1559) (16.3277, 8.1143) knots 0 0 0 0 1 1 1 1
  spline S996 degree 3 poles (16.3277, 8.1143) (16.2085, 8.0505) (16.1862, 7.9684) (16.1862, 7.5946) knots 0 0 0 0 1 1 1 1
  spline S997 degree 3 poles (16.1862, 7.5946) (16.1862, 7.2671) (16.2166, 7.1254) (16.3019, 7.0545) knots 0 0 0 0 1 1 1 1
  spline S998 degree 3 poles (16.3019, 7.0545) (16.395, 6.9772) (17.0744, 6.9513) (19.7846, 6.9221) knots 0 0 0 0 1 1 1 1
  spline S999 degree 3 poles (19.7846, 6.9221) (21.6365, 6.9021) (23.2837, 6.8785) (23.4452, 6.8696) knots 0 0 0 0 1 1 1 1
  spline S1000 degree 3 poles (23.4452, 6.8696) (23.6716, 6.8571) (23.7613, 6.8856) (23.8373, 6.9942) knots 0 0 0 0 1 1 1 1
  spline S1001 degree 3 poles (-15.7358, 7.3278) (-15.1294, 7.5456) (-14.1698, 8.0084) (-14.0684, 8.1319) knots 0 0 0 0 1 1 1 1
  spline S1002 degree 3 poles (-14.0684, 8.1319) (-13.9914, 8.2258) (-14.0004, 8.358) (-14.1234, 8.9315) knots 0 0 0 0 1 1 1 1
  spline S1003 degree 3 poles (-14.1234, 8.9315) (-14.2044, 9.3094) (-14.2869, 9.6721) (-14.3068, 9.7375) knots 0 0 0 0 1 1 1 1
  spline S1004 degree 3 poles (-14.3068, 9.7375) (-14.3687, 9.9415) (-14.5966, 9.9509) (-15.0534, 9.7683) knots 0 0 0 0 1 1 1 1
  spline S1005 degree 3 poles (-15.0534, 9.7683) (-15.294, 9.6722) (-15.7113, 9.5399) (-15.9808, 9.4743) knots 0 0 0 0 1 1 1 1
  spline S1006 degree 3 poles (-15.9808, 9.4743) (-16.2503, 9.4087) (-16.5084, 9.3198) (-16.5543, 9.2768) knots 0 0 0 0 1 1 1 1
  spline S1007 degree 3 poles (-16.5543, 9.2768) (-16.6002, 9.2337) (-16.7791, 8.7419) (-16.952, 8.1837) knots 0 0 0 0 1 1 1 1
  spline S1008 degree 3 poles (-16.952, 8.1837) (-17.2322, 7.2791) (-17.255, 7.1564) (-17.1624, 7.0541) knots 0 0 0 0 1 1 1 1
  spline S1009 degree 3 poles (-17.1624, 7.0541) (-17.0662, 6.9477) (-17.0239, 6.9485) (-16.5897, 7.0644) knots 0 0 0 0 1 1 1 1
  spline S1010 degree 3 poles (-16.5897, 7.0644) (-16.3318, 7.1332) (-15.9476, 7.2517) (-15.7358, 7.3278) knots 0 0 0 0 1 1 1 1
  spline S1011 degree 3 poles (10.7818, 7.3574) (10.828, 7.4036) (10.8658, 7.5706) (10.8658, 7.7285) knots 0 0 0 0 1 1 1 1
  spline S1012 degree 3 poles (10.8658, 7.7285) (10.8658, 7.8863) (10.828, 8.0533) (10.7818, 8.0995) knots 0 0 0 0 1 1 1 1
  spline S1013 degree 3 poles (10.7818, 8.0995) (10.7293, 8.152) (10.4681, 8.1835) (10.0842, 8.1835) knots 0 0 0 0 1 1 1 1
  spline S1014 degree 3 poles (10.0842, 8.1835) (9.4977, 8.1835) (9.4597, 8.1931) (9.2232, 8.4008) knots 0 0 0 0 1 1 1 1
  spline S1015 degree 3 poles (9.2232, 8.4008) (9.0209, 8.5783) (8.9757, 8.6669) (8.9757, 8.8858) knots 0 0 0 0 1 1 1 1
  spline S1016 degree 3 poles (8.9757, 8.8858) (8.9757, 9.3814) (9.0139, 9.3736) (6.5963, 9.3736) knots 0 0 0 0 1 1 1 1
  spline S1017 degree 3 poles (6.5963, 9.3736) (5.4086, 9.3736) (4.3871, 9.3544) (4.3262, 9.3311) knots 0 0 0 0 1 1 1 1
  spline S1018 degree 3 poles (4.3262, 9.3311) (4.1588, 9.2668) (4.1632, 7.5872) (4.3313, 7.4015) knots 0 0 0 0 1 1 1 1
  spline S1019 degree 3 poles (4.3313, 7.4015) (4.4402, 7.2811) (4.6336, 7.2734) (7.5725, 7.2734) knots 0 0 0 0 1 1 1 1
  spline S1020 degree 3 poles (7.5725, 7.2734) (9.91, 7.2734) (10.719, 7.2946) (10.7818, 7.3574) knots 0 0 0 0 1 1 1 1
  spline S1021 degree 3 poles (-31.0386, 8.5304) (-30.2287, 8.5745) (-29.8268, 8.6238) (-29.7649, 8.6867) knots 0 0 0 0 1 1 1 1
  spline S1022 degree 3 poles (-29.7649, 8.6867) (-29.7152, 8.7372) (-29.5163, 9.3992) (-29.323, 10.1577) knots 0 0 0 0 1 1 1 1
  spline S1023 degree 3 poles (-29.323, 10.1577) (-28.9482, 11.628) (-28.3029, 13.6457) (-27.8834, 14.6592) knots 0 0 0 0 1 1 1 1
  spline S1024 degree 3 poles (-27.8834, 14.6592) (-27.6374, 15.2534) (-27.6326, 15.2809) (-27.7547, 15.3972) knots 0 0 0 0 1 1 1 1
  spline S1025 degree 3 poles (-27.7547, 15.3972) (-27.8718, 15.5086) (-27.9428, 15.5107) (-28.6801, 15.4238) knots 0 0 0 0 1 1 1 1
  spline S1026 degree 3 poles (-28.6801, 15.4238) (-29.7883, 15.2931) (-30.5216, 15.1317) (-30.653, 14.9894) knots 0 0 0 0 1 1 1 1
  spline S1027 degree 3 poles (-30.653, 14.9894) (-30.9725, 14.6434) (-32.0857, 11.7359) (-32.6407, 9.7976) knots 0 0 0 0 1 1 1 1
  spline S1028 degree 3 poles (-32.6407, 9.7976) (-32.9437, 8.7394) (-32.9585, 8.6513) (-32.8523, 8.534) knots 0 0 0 0 1 1 1 1
  spline S1029 degree 3 poles (-32.8523, 8.534) (-32.7699, 8.443) (-32.6666, 8.416) (-32.48, 8.437) knots 0 0 0 0 1 1 1 1
  spline S1030 degree 3 poles (-32.48, 8.437) (-32.338, 8.4529) (-31.6894, 8.495) (-31.0386, 8.5304) knots 0 0 0 0 1 1 1 1
  spline S1031 degree 3 poles (-25.6351, 8.7358) (-25.1104, 8.743) (-25.0633, 8.7557) (-24.993, 8.9099) knots 0 0 0 0 1 1 1 1
  spline S1032 degree 3 poles (-24.993, 8.9099) (-24.944, 9.0174) (-24.9412, 9.1004) (-24.9851, 9.1442) knots 0 0 0 0 1 1 1 1
  spline S1033 degree 3 poles (-24.9851, 9.1442) (-25.1212, 9.2804) (-25.5937, 10.4749) (-25.7541, 11.0887) knots 0 0 0 0 1 1 1 1
  spline S1034 degree 3 poles (-25.7541, 11.0887) (-25.8985, 11.6411) (-25.9188, 11.8783) (-25.9184, 13.0138) knots 0 0 0 0 1 1 1 1
  spline S1035 degree 3 poles (-25.9184, 13.0138) (-25.9181, 13.9985) (-25.8877, 14.4482) (-25.7918, 14.8902) knots 0 0 0 0 1 1 1 1
  spline S1036 degree 3 poles (-25.7918, 14.8902) (-25.6929, 15.3461) (-25.6838, 15.4934) (-25.7496, 15.5728) knots 0 0 0 0 1 1 1 1
  spline S1037 degree 3 poles (-25.7496, 15.5728) (-25.8543, 15.699) (-26.4452, 15.7084) (-26.6026, 15.5864) knots 0 0 0 0 1 1 1 1
  spline S1038 degree 3 poles (-26.6026, 15.5864) (-26.9087, 15.3492) (-28.0708, 12.017) (-28.617, 9.8103) knots 0 0 0 0 1 1 1 1
  spline S1039 degree 3 poles (-28.617, 9.8103) (-28.9268, 8.5589) (-28.9971, 8.6249) (-27.4142, 8.6833) knots 0 0 0 0 1 1 1 1
  spline S1040 degree 3 poles (-27.4142, 8.6833) (-26.7472, 8.7079) (-25.9466, 8.7315) (-25.6351, 8.7358) knots 0 0 0 0 1 1 1 1
  spline S1041 degree 3 poles (-12.3099, 9.2503) (-11.0991, 10.167) (-9.5151, 11.8734) (-9.6067, 12.1622) knots 0 0 0 0 1 1 1 1
  spline S1042 degree 3 poles (-9.6067, 12.1622) (-9.6376, 12.2593) (-9.8394, 12.3565) (-10.3394, 12.515) knots 0 0 0 0 1 1 1 1
  spline S1043 degree 3 poles (-10.3394, 12.515) (-10.719, 12.6353) (-11.0733, 12.7338) (-11.1267, 12.7338) knots 0 0 0 0 1 1 1 1
  spline S1044 degree 3 poles (-11.1267, 12.7338) (-11.1802, 12.7338) (-11.4239, 12.4989) (-11.6683, 12.2118) knots 0 0 0 0 1 1 1 1
  spline S1045 degree 3 poles (-11.6683, 12.2118) (-12.1403, 11.6573) (-12.6674, 11.1736) (-13.2681, 10.7436) knots 0 0 0 0 1 1 1 1
  spline S1046 degree 3 poles (-13.2681, 10.7436) (-13.4819, 10.5906) (-13.6357, 10.4269) (-13.6357, 10.3523) knots 0 0 0 0 1 1 1 1
  spline S1047 degree 3 poles (-13.6357, 10.3523) (-13.6357, 10.137) (-13.3429, 8.9242) (-13.2684, 8.831) knots 0 0 0 0 1 1 1 1
  spline S1048 degree 3 poles (-13.2684, 8.831) (-13.1406, 8.6711) (-12.9849, 8.7393) (-12.3099, 9.2503) knots 0 0 0 0 1 1 1 1
  spline S1049 degree 3 poles (16.1528, 9.0002) (16.2466, 9.0939) (16.2604, 9.1933) (16.2232, 9.5077) knots 0 0 0 0 1 1 1 1
  spline S1050 degree 3 poles (16.2232, 9.5077) (16.1176, 10.4024) (15.8293, 11.9927) (15.7569, 12.0799) knots 0 0 0 0 1 1 1 1
  spline S1051 degree 3 poles (15.7569, 12.0799) (15.7037, 12.1439) (15.5026, 12.1737) (15.1235, 12.1737) knots 0 0 0 0 1 1 1 1
  spline S1052 degree 3 poles (15.1235, 12.1737) (14.818, 12.1737) (14.4281, 12.209) (14.2571, 12.252) knots 0 0 0 0 1 1 1 1
  spline S1053 degree 3 poles (14.2571, 12.252) (13.9652, 12.3255) (13.946, 12.3451) (13.946, 12.5688) knots 0 0 0 0 1 1 1 1
  spline S1054 degree 3 poles (13.946, 12.5688) (13.946, 12.8769) (14.1124, 12.9438) (14.8788, 12.9438) knots 0 0 0 0 1 1 1 1
  spline S1055 degree 3 poles (14.8788, 12.9438) (15.682, 12.9438) (15.6778, 12.9324) (15.3743, 14.2825) knots 0 0 0 0 1 1 1 1
  spline S1056 degree 3 poles (15.3743, 14.2825) (15.2413, 14.8745) (15.0998, 15.5054) (15.0599, 15.6845) knots 0 0 0 0 1 1 1 1
  spline S1057 degree 3 poles (15.0599, 15.6845) (14.9397, 16.2248) (14.9949, 16.2108) (12.791, 16.2597) knots 0 0 0 0 1 1 1 1
  spline S1058 degree 3 poles (12.791, 16.2597) (9.6171, 16.33) (-2.3896, 16.4006) (-2.5909, 16.35) knots 0 0 0 0 1 1 1 1
  spline S1059 degree 3 poles (-2.5909, 16.35) (-2.6925, 16.3245) (-2.7923, 16.2486) (-2.8127, 16.1813) knots 0 0 0 0 1 1 1 1
  spline S1060 degree 3 poles (-2.8127, 16.1813) (-2.8567, 16.0361) (-2.9634, 13.9564) (-3.0681, 11.206) knots 0 0 0 0 1 1 1 1
  spline S1061 degree 3 poles (-3.0681, 11.206) (-3.1258, 9.6883) (-3.1241, 9.1997) (-3.0607, 9.1233) knots 0 0 0 0 1 1 1 1
  spline S1062 degree 3 poles (-3.0607, 9.1233) (-2.9326, 8.969) (3.2479, 8.9749) (3.3762, 9.1296) knots 0 0 0 0 1 1 1 1
  spline S1063 degree 3 poles (3.3762, 9.1296) (3.4425, 9.2094) (3.4522, 9.4474) (3.4154, 10.0934) knots 0 0 0 0 1 1 1 1
  spline S1064 degree 3 poles (3.4154, 10.0934) (3.3596, 11.0728) (3.4088, 11.2918) (3.7013, 11.3652) knots 0 0 0 0 1 1 1 1
  spline S1065 degree 3 poles (3.7013, 11.3652) (3.9838, 11.4361) (4.1454, 11.2137) (4.1454, 10.7539) knots 0 0 0 0 1 1 1 1
  spline S1066 degree 3 poles (4.1454, 10.7539) (4.1454, 10.1199) (4.0511, 10.1436) (6.569, 10.1436) knots 0 0 0 0 1 1 1 1
  spline S1067 degree 3 poles (6.569, 10.1436) (8.71, 10.1436) (8.7626, 10.147) (8.8379, 10.2877) knots 0 0 0 0 1 1 1 1
  spline S1068 degree 3 poles (8.8379, 10.2877) (8.8803, 10.367) (8.8947, 10.5246) (8.8698, 10.6381) knots 0 0 0 0 1 1 1 1
  spline S1069 degree 3 poles (8.8698, 10.6381) (8.8331, 10.8048) (8.8684, 10.8999) (9.0545, 11.1348) knots 0 0 0 0 1 1 1 1
  line L131 (9.0545, 11.1348) -> (9.2846, 11.4253)
  line L132 (9.2846, 11.4253) -> (10.9851, 11.3817)
  spline S1070 degree 3 poles (10.9851, 11.3817) (13.2214, 11.3244) (13.1142, 11.3906) (13.2801, 9.9643) knots 0 0 0 0 1 1 1 1
  spline S1071 degree 3 poles (13.2801, 9.9643) (13.3316, 9.5206) (13.4109, 9.1129) (13.4561, 9.0584) knots 0 0 0 0 1 1 1 1
  spline S1072 degree 3 poles (13.4561, 9.0584) (13.5408, 8.9564) (13.8956, 8.9259) (15.3236, 8.8976) knots 0 0 0 0 1 1 1 1
  spline S1073 degree 3 poles (15.3236, 8.8976) (15.9081, 8.8861) (16.0571, 8.9045) (16.1528, 9.0002) knots 0 0 0 0 1 1 1 1
  spline S1074 degree 3 poles (-3.9976, 9.1112) (-3.9363, 9.1726) (-3.889, 9.7502) (-3.8384, 11.0537) knots 0 0 0 0 1 1 1 1
  spline S1075 degree 3 poles (-3.8384, 11.0537) (-3.7989, 12.074) (-3.7304, 13.6407) (-3.6864, 14.5354) knots 0 0 0 0 1 1 1 1
  spline S1076 degree 3 poles (-3.6864, 14.5354) (-3.6224, 15.8328) (-3.624, 16.1834) (-3.6942, 16.268) knots 0 0 0 0 1 1 1 1
  spline S1077 degree 3 poles (-3.6942, 16.268) (-3.7673, 16.3561) (-4.0087, 16.3736) (-5.1212, 16.3718) knots 0 0 0 0 1 1 1 1
  spline S1078 degree 3 poles (-5.1212, 16.3718) (-6.0647, 16.3702) (-6.4934, 16.3443) (-6.5725, 16.284) knots 0 0 0 0 1 1 1 1
  spline S1079 degree 3 poles (-6.5725, 16.284) (-6.6342, 16.237) (-6.7674, 15.9359) (-6.8684, 15.6149) knots 0 0 0 0 1 1 1 1
  spline S1080 degree 3 poles (-6.8684, 15.6149) (-7.527, 13.5226) (-8.6954, 11.6349) (-10.3907, 9.9242) knots 0 0 0 0 1 1 1 1
  spline S1081 degree 3 poles (-10.3907, 9.9242) (-11.0083, 9.3009) (-11.0527, 9.2378) (-10.9751, 9.0929) knots 0 0 0 0 1 1 1 1
  line L133 (-10.9751, 9.0929) -> (-10.8912, 8.936)
  line L134 (-10.8912, 8.936) -> (-7.488, 8.9799)
  spline S1082 degree 3 poles (-7.488, 8.9799) (-4.9106, 9.0132) (-4.0636, 9.045) (-3.9976, 9.1112) knots 0 0 0 0 1 1 1 1
  spline S1083 degree 3 poles (-16.7809, 10.1633) (-16.6681, 10.2508) (-16.3988, 11.1622) (-16.1559, 12.2787) knots 0 0 0 0 1 1 1 1
  spline S1084 degree 3 poles (-16.1559, 12.2787) (-15.9859, 13.06) (-15.9855, 13.1012) (-16.1459, 13.2013) knots 0 0 0 0 1 1 1 1
  spline S1085 degree 3 poles (-16.1459, 13.2013) (-16.2593, 13.2722) (-16.3696, 13.1959) (-17.0082, 12.6056) knots 0 0 0 0 1 1 1 1
  spline S1086 degree 3 poles (-17.0082, 12.6056) (-17.4109, 12.2333) (-18.0612, 11.6639) (-18.4532, 11.3402) knots 0 0 0 0 1 1 1 1
  spline S1087 degree 3 poles (-18.4532, 11.3402) (-19.1986, 10.7249) (-19.2858, 10.5753) (-19.006, 10.392) knots 0 0 0 0 1 1 1 1
  spline S1088 degree 3 poles (-19.006, 10.392) (-18.6015, 10.127) (-17.0353, 9.966) (-16.7809, 10.1633) knots 0 0 0 0 1 1 1 1
  spline S1089 degree 3 poles (-15.0521, 10.5966) (-14.8493, 10.691) (-14.664, 10.8189) (-14.6402, 10.8808) knots 0 0 0 0 1 1 1 1
  spline S1090 degree 3 poles (-14.6402, 10.8808) (-14.5978, 10.9913) (-14.8535, 12.0911) (-14.9775, 12.3312) knots 0 0 0 0 1 1 1 1
  spline S1091 degree 3 poles (-14.9775, 12.3312) (-15.0919, 12.5531) (-15.3034, 12.4796) (-15.3807, 12.1912) knots 0 0 0 0 1 1 1 1
  spline S1092 degree 3 poles (-15.3807, 12.1912) (-15.6525, 11.1759) (-15.7462, 10.6255) (-15.664, 10.5265) knots 0 0 0 0 1 1 1 1
  spline S1093 degree 3 poles (-15.664, 10.5265) (-15.5494, 10.3884) (-15.4829, 10.3961) (-15.0521, 10.5966) knots 0 0 0 0 1 1 1 1
  spline S1094 degree 3 poles (23.1913, 10.6743) (23.2665, 10.7649) (23.2672, 10.876) (23.1949, 11.2868) knots 0 0 0 0 1 1 1 1
  spline S1095 degree 3 poles (23.1949, 11.2868) (23.1463, 11.5629) (23.0895, 11.8877) (23.0687, 12.0086) knots 0 0 0 0 1 1 1 1
  spline S1096 degree 3 poles (23.0687, 12.0086) (23.0375, 12.1896) (23.0725, 12.2735) (23.2662, 12.4827) knots 0 0 0 0 1 1 1 1
  line L135 (23.2662, 12.4827) -> (23.5016, 12.7368)
  line L136 (23.5016, 12.7368) -> (24.7617, 12.6744)
  spline S1097 degree 3 poles (24.7617, 12.6744) (25.868, 12.6195) (26.0372, 12.6253) (26.1483, 12.7223) knots 0 0 0 0 1 1 1 1
  spline S1098 degree 3 poles (26.1483, 12.7223) (26.2361, 12.7989) (26.2614, 12.8858) (26.2311, 13.0067) knots 0 0 0 0 1 1 1 1
  spline S1099 degree 3 poles (26.2311, 13.0067) (26.1143, 13.4718) (25.2601, 15.643) (25.1671, 15.711) knots 0 0 0 0 1 1 1 1
  spline S1100 degree 3 poles (25.1671, 15.711) (25.1087, 15.7537) (24.9149, 15.7948) (24.7363, 15.8024) knots 0 0 0 0 1 1 1 1
  spline S1101 degree 3 poles (24.7363, 15.8024) (24.5578, 15.81) (23.9077, 15.8459) (23.2916, 15.8821) knots 0 0 0 0 1 1 1 1
  spline S1102 degree 3 poles (23.2916, 15.8821) (22.6756, 15.9184) (21.6833, 15.9663) (21.0865, 15.9887) knots 0 0 0 0 1 1 1 1
  spline S1103 degree 3 poles (21.0865, 15.9887) (20.4897, 16.011) (19.3084, 16.0593) (18.4613, 16.096) knots 0 0 0 0 1 1 1 1
  spline S1104 degree 3 poles (18.4613, 16.096) (17.6143, 16.1326) (16.7004, 16.163) (16.4305, 16.1633) knots 0 0 0 0 1 1 1 1
  spline S1105 degree 3 poles (16.4305, 16.1633) (15.7743, 16.1642) (15.7334, 16.1003) (15.9131, 15.3533) knots 0 0 0 0 1 1 1 1
  spline S1106 degree 3 poles (15.9131, 15.3533) (15.9865, 15.0484) (16.1248, 14.4209) (16.2204, 13.9588) knots 0 0 0 0 1 1 1 1
  spline S1107 degree 3 poles (16.2204, 13.9588) (16.4515, 12.8428) (16.4096, 12.8738) (17.6878, 12.8738) knots 0 0 0 0 1 1 1 1
  spline S1108 degree 3 poles (17.6878, 12.8738) (18.2356, 12.8738) (19.3111, 12.8529) (20.0777, 12.8275) knots 0 0 0 0 1 1 1 1
  line L137 (20.0777, 12.8275) -> (21.4715, 12.7812)
  line L138 (21.4715, 12.7812) -> (21.6855, 12.565)
  spline S1109 degree 3 poles (21.6855, 12.565) (21.8636, 12.3851) (21.9262, 12.225) (22.0578, 11.6137) knots 0 0 0 0 1 1 1 1
  spline S1110 degree 3 poles (22.0578, 11.6137) (22.2891, 10.5387) (22.2733, 10.5636) (22.7215, 10.5636) knots 0 0 0 0 1 1 1 1